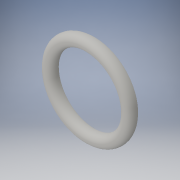
# Autodesk Inventor part: cw O-ring
Saved by Autodesk Inventor 2016 (Build 200138000, 138)
## iProperties
Created: 2017-09-08
Part Number: cw O-ring
Material: Generic
Document SubType Name: Modeling
Designer: student
Density: 1 g/cm^3
Appearance: Default
Author: student
Autodesk Inventor part; units mm, degrees
ref_plane "YZ Plane" through (0, 0, 0) normal (1, 0, 0) x (0, 1, 0)
ref_plane "XZ Plane" through (0, 0, 0) normal (0, 1, 0) x (-1, 0, 0)
ref_plane "XY Plane" through (0, 0, 0) normal (0, 0, 1) x (1, 0, 0)
sketch "Sketch1" plane through (0, 0, 0) normal (0, 0, 1) x (1, 0, 0)
  circle A0 centre (0, 0) radius 19.3421
  circle A1 centre (0, 0) radius 14.2621
  dimension "d0" = 38.6842
  dimension "d8" = 28.5242
  constraints: 2 centre point, 2 coincident
  measures "d0" diameter of A0
  measures "d8" diameter of A1
sketch "Sketch4" plane through (0, 0, 0) normal (1, 0, 0) x (0, 1, 0)
  circle A0 centre (16.8256, 0) radius 2.54
  point P0 (0, 0)
  dimension "d9" = 5.08
  constraints: 1 centre point
  measures "d9" diameter of A0
sweep "Sweep1" add profiles "Sketch4" path "Sketch1" path curves A0
body "Solid2"
